Housing_v12 (Autodesk Fusion 360 design; units mm, degrees)
Autodesk Fusion 360 part; units mm, degrees
sketch "Sketch1" plane through (0, 0, 0) normal (0, 0, 1) x (1, 0, 0)
  circle A0 centre (0, 0) radius 65
  circle A1 centre (0, 0) radius 61.375 construction
  circle A2 centre (0, 61.375) radius 1.5
  circle A3 centre (0, 0) radius 42.5
  dimension "d1" = 130
  dimension "d2" = 122.75
  dimension "d3" = 3
  dimension "LargeBearingDia" = 85
  constraint coincident A0.centre A1.centre
  constraint coincident A1 A2.centre
  constraint concentric A1 A3
  measures "d1" diameter of A0
  measures "d2" diameter of A1
  measures "d3" diameter of A2
  measures "LargeBearingDia" diameter of A3
extrude "Extrude1" add sketch "Sketch1" along normal blind 10 contours A0 | A2
extrude "Extrude2" cut sketch "Sketch1" along normal blind 7 contours A2
pattern_circular "C-Pattern1" count 6 over 360 about axis through (0, 0, 1.75) along (0, 0, 1) of "Extrude2"
sketch "Sketch2" plane through (0, 0, 10) normal (0, 0, 1) x (-1, 0, 0)
  circle A0 centre (0, 0) radius 42.5
  circle A1 centre (0, 0) radius 65
  circle A2 centre (0, 0) radius 52.5 construction
  circle A3 centre (0, -52.5) radius 7.05
  circle A4 centre (28.3836, -44.1658) radius 7.05
  circle A5 centre (47.7557, -21.8093) radius 7.05
  circle A6 centre (51.9656, 7.4715) radius 7.05
  circle A7 centre (39.6769, 34.3802) radius 7.05
  circle A8 centre (14.791, 50.3734) radius 7.05
  circle A9 centre (-14.791, 50.3734) radius 7.05
  circle A10 centre (-39.6769, 34.3802) radius 7.05
  circle A11 centre (-51.9656, 7.4715) radius 7.05
  circle A12 centre (-47.7557, -21.8093) radius 7.05
  circle A13 centre (-28.3836, -44.1658) radius 7.05
  circle A14 centre (0, 0) radius 56.5
  dimension "d11" = 105
  dimension "d12" = 14.1
  dimension "d14" = 360
  dimension "d15" = 113
  constraint coincident A0.centre A1.centre
  constraint coincident A2 A3.centre
  measures "d11" diameter of A2
  measures "d12" diameter of A3
  measures "d15" diameter of A14
extrude "Extrude3" add sketch "Sketch2" along normal blind 17.5 contours A1
extrude "Extrude4" add 1 faces at (57.7924, -22.5756, 27.5) along direction (0, 0, 1) blind 1.75
sketch "Sketch3" plane through (0, 0, 29.25) normal (0, 0, 1) x (-1, 0, 0)
  arc A0 (53.6005, -17.8672) -> (56.4631, 2.0424) centre (0, 0) ccw
  arc A1 (48.604, -28.8081) -> (53.6005, -17.8672) centre (47.7557, -21.8093) ccw
  arc A2 (35.4319, -44.0094) -> (48.604, -28.8081) centre (0, 0) ccw
  arc A3 (25.3134, -50.5122) -> (35.4319, -44.0094) centre (28.3836, -44.1658) ccw
  arc A4 (6.0139, -56.179) -> (25.3134, -50.5122) centre (0, 0) ccw
  arc A5 (-6.0139, -56.179) -> (6.0139, -56.179) centre (0, -52.5) ccw
  arc A6 (-25.3134, -50.5122) -> (-6.0139, -56.179) centre (0, 0) ccw
  arc A7 (-35.4319, -44.0094) -> (-25.3134, -50.5122) centre (-28.3836, -44.1658) ccw
  arc A8 (-48.604, -28.8081) -> (-35.4319, -44.0094) centre (0, 0) ccw
  arc A9 (-53.6005, -17.8672) -> (-48.604, -28.8081) centre (-47.7557, -21.8093) ccw
  arc A10 (-56.4631, 2.0424) -> (-53.6005, -17.8672) centre (0, 0) ccw
  arc A11 (-54.7513, 13.9478) -> (-56.4631, 2.0424) centre (-51.9656, 7.4715) ccw
  arc A12 (-46.3956, 32.2444) -> (-54.7513, 13.9478) centre (0, 0) ccw
  arc A13 (-38.519, 41.3345) -> (-46.3956, 32.2444) centre (-39.6769, 34.3802) ccw
  arc A14 (-21.5978, 52.2091) -> (-38.519, 41.3345) centre (0, 0) ccw
  arc A15 (-10.0571, 55.5977) -> (-21.5978, 52.2091) centre (-14.791, 50.3734) ccw
  arc A16 (10.0571, 55.5977) -> (-10.0571, 55.5977) centre (0, 0) ccw
  arc A17 (21.5978, 52.2091) -> (10.0571, 55.5977) centre (14.791, 50.3734) ccw
  arc A18 (38.519, 41.3345) -> (21.5978, 52.2091) centre (0, 0) ccw
  arc A19 (46.3956, 32.2444) -> (38.519, 41.3345) centre (39.6769, 34.3802) ccw
  arc A20 (54.7513, 13.9478) -> (46.3956, 32.2444) centre (0, 0) ccw
  arc A21 (56.4631, 2.0424) -> (54.7513, 13.9478) centre (51.9656, 7.4715) ccw
  circle A22 centre (0, 0) radius 65
  circle A23 centre (0, 0) radius 61.0224 construction
  circle A24 centre (0, -61.0224) radius 1.5
  circle A25 centre (52.847, -30.5112) radius 1.5
  circle A26 centre (52.847, 30.5112) radius 1.5
  circle A27 centre (0, 61.0224) radius 1.5
  circle A28 centre (-52.847, 30.5112) radius 1.5
  circle A29 centre (-52.847, -30.5112) radius 1.5
  dimension "d20" = 3
  dimension "d22" = 360
  dimension "d25" = 122.0449
  constraint concentric A0 A23
  constraint coincident A23 A24.centre
  measures "d20" diameter of A24
  measures "d25" diameter of A23
extrude "Extrude5" cut sketch "Sketch3" against normal blind 10 contours A5 A24 | A25 | A26 | A27 | A28 | A29 picked at (0.0626, -61.5282)
equation "d3 = ScrewDia_3mm"
equation "d20 = ScrewDia_3mm"
equation "ScrewDia_3mm = 3 mm"
